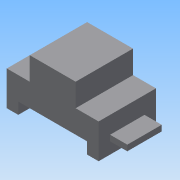
# Autodesk Inventor part: Part1
Saved by Autodesk Inventor 2015 (Build 190159000, 159)
## iProperties
Created: 2016-10-27
Part Number: Part1
Material: Generic
Document SubType Name: Modeling
Designer: Aniket Pant
Density: 1 g/cm^3
Appearance: Default
Author: Aniket Pant
Autodesk Inventor part; units mm, degrees
ref_plane "YZ Plane" through (0, 0, 0) normal (1, 0, 0) x (0, 1, 0)
ref_plane "XZ Plane" through (0, 0, 0) normal (0, 1, 0) x (-1, 0, 0)
ref_plane "XY Plane" through (0, 0, 0) normal (0, 0, 1) x (1, 0, 0)
sketch "Sketch1" plane through (0, 0, 0) normal (0, 0, 1) x (1, 0, 0)
  line L0 (0, 0) -> (0, 38.1)
  line L1 (0, 38.1) -> (25.4, 38.1)
  line L2 (25.4, 38.1) -> (25.4, 63.5)
  line L3 (25.4, 63.5) -> (76.2, 63.5)
  line L4 (76.2, 63.5) -> (76.2, 38.1)
  line L5 (76.2, 38.1) -> (101.6, 38.1)
  line L6 (101.6, 38.1) -> (101.6, 0)
  line L7 (101.6, 0) -> (88.9, 0)
  line L8 (88.9, 0) -> (88.9, 12.7)
  line L9 (88.9, 12.7) -> (12.7, 12.7)
  line L10 (12.7, 12.7) -> (12.7, 0)
  line L11 (12.7, 0) -> (0, 0)
  dimension "d0" = 38.1
  dimension "d1" = 25.4
  dimension "d2" = 25.4
  dimension "d3" = 50.8
  dimension "d4" = 25.4
  dimension "d5" = 38.1
  dimension "d6" = 12.7
  dimension "d7" = 12.7
  dimension "d8" = 76.2
  constraints: 24 end point, 7 perpendicular, 3 point on line, 2 vertical, 1 horizontal
  measures "d0" distance of L0.start L0.end
  measures "d1" distance of L0.end L1.end
  measures "d2" distance of L1.end L2.end
  measures "d3" distance of L2.end L3.end
  measures "d4" distance of L4.end L5.end
  measures "d5" distance of L5.end L6.end
  measures "d6" distance of L6.end L7.end
  measures "d7" distance of L7.end L8.end
  measures "d8" distance of L8.end L9.end
extrude "Extrusion1" add sketch "Sketch1" along normal blind 63.5
sketch "Sketch2" plane through (101.6, 0, 0) normal (1, 0, 0) x (0, 0, -1)
  point P0 (0, 0)
sketch "Sketch3" plane through (101.6, 0, 0) normal (1, 0, 0) x (0, 0, -1)
  point P0 (0, 0)
sketch "Sketch4" plane through (101.6, 0, 0) normal (1, 0, 0) x (0, 0, -1)
  line L0 (0, 12.7) -> (-63.5, 12.7) projected
  line L1 (-50.8, 12.7) -> (-12.7, 12.7)
  line L2 (-12.7, 12.7) -> (-12.7, 19.05)
  line L3 (-12.7, 19.05) -> (-50.8, 19.05)
  line L4 (-50.8, 19.05) -> (-50.8, 12.7)
  line L5 (-63.5, 0) -> (-63.5, 38.1) projected
  point P0 (0, 0)
  dimension "d11" = 38.1
  dimension "d12" = 6.35
  dimension "d13" = 12.7
  constraints: 8 end point, 2 parallel, 1 horizontal, 1 perpendicular, 1 point on line
  measures "d11" distance of L3.end L2.end
  measures "d12" distance of L1.end L2.end
  measures "d13" distance between parallel lines of L5 L4
extrude "Extrusion2" add sketch "Sketch4" along normal blind 19.05
body "Solid1"
